Autodesk Inventor part; units mm, degrees
(part 2 of 2)
sketch "Szkic26" plane through (-1.315511, 25.101441, 20) normal (0, 0, -1) x (-1, 0, 0)
  circle A0 centre (0, 0) radius 24.95
  circle A1 centre (-9.295869, 14.314383) radius 2
  circle A2 centre (17.044553, 0.893267) radius 2
  circle A3 centre (-7.748685, -15.20765) radius 2
  circle A4 centre (-17.044553, -0.893267) radius 2
  circle A5 centre (9.295869, -14.314383) radius 2
  circle A6 centre (7.748685, 15.20765) radius 2
  circle A7 centre (0, 0) radius 8
  circle A8 centre (-17.044553, -0.893267) radius 2
  circle A9 centre (-17.044553, -0.893267) radius 2.25
  circle A10 centre (-7.748685, -15.20765) radius 2.25
  circle A11 centre (9.295869, -14.314383) radius 2.25
  circle A12 centre (17.044553, 0.893267) radius 2.25
  circle A13 centre (7.748685, 15.20765) radius 2.25
  circle A14 centre (-9.295869, 14.314383) radius 2.25
  point P0 (-1.315511, -25.101441)
  dimension "d139" = 4.5
  dimension "d142" = 360
  constraints: 6 centre point, 1 coincident, 13 other
  measures "d139" diameter of A9
extrude "Wyciągnięcie proste28" cut sketch "Szkic26" against normal through all contours A1 | A2 | A3 | A4 | A5 | A6 | A9 | A10 | A11 | A12 | A13 | A14
fillet "Zaokrąglenie6" radius 2 1 edges at (-71.3155, 25.1014, 27)
fillet "Zaokrąglenie7" radius 0.5 1 edges at (-71.3155, 25.1014, 42)
chamfer "Faza4" distance 1 angle 45 6 edges at (-6.8142, 40.3091, 20) (-16.1101, 25.9947, 20) (-8.3614, 10.7871, 20) (8.6832, 9.8938, 20) (17.979, 24.2082, 20) (10.2304, 39.4158, 20)
body "Solid1"
